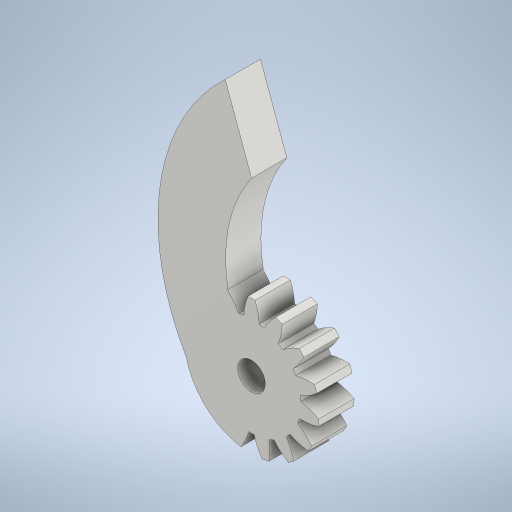
# Autodesk Inventor part: Spur Gear1
Saved by Autodesk Inventor 2024 (Build 280153000, 153)
## iProperties
CustomPartVersion: 1
Created: 2023-09-24
Part Number: Spur Gear1
Material: Steel
Document SubType Name: Modeling
Designer: jebes windows
Categories: <?xml version="1.0" encoding="UTF-16"?> <MemberInstance><Categories><FamilyTemplate><FamilyTemplateParameter ValueType="xs:double" Id="1" ObjectReferenceKey="da_z" ObjectType="kUserParameterObject"/><FamilyTemplateParameter ValueType="xs:double" Id="2" ObjectReferenceKey="da_b" ObjectType="kUserParameterObject"/><FamilyTemplateParameter ValueType="xs:double" Id="3" ObjectReferenceKey="da_beta" ObjectType="kUserParameterObject"/><FamilyTemplateParameter ValueType="xs:double" Id="4" ObjectReferenceKey="da_da" ObjectType="kUserParameterObject"/><FamilyTemplateParameter ValueType="xs:double" Id="5" ObjectReferenceKey="da_aw" ObjectType="kUserParameterObject"/><FamilyTemplateParameter ValueType="xs:string" Id="6" ObjectReferenceKey="EAIAABAAAACIAQAAAAAAAIAAAAAAAAAA" ObjectType="83910656" SubObjectId="SurfaceGeometry"/></FamilyTemplate><ParamToTemplateMap><ParamToTemplate CategoryParameter="//CategoryParameter[@InternalName='046C89C9-8512-4d59-83FE-43B91F4F132A']" TemplateParameter="1"/><ParamToTemplate CategoryParameter="//CategoryParameter[@InternalName='2552DF32-E462-4b46-AEBF-C6C7768E72AC']" TemplateParameter="2"/><ParamToTemplate CategoryParameter="//CategoryParameter[@InternalName='C9EE641D-15FC-4fae-A226-E94C4372FDD7']" TemplateParameter="3"/><ParamToTemplate><ParamToTemplate CategoryParameter="//CategoryParameter[@InternalName='00B6519A-459B-49c7-AD84-2E56D39A5744']" ConstantValue="0.000000"/></ParamToTemplate><ParamToTemplate><ParamToTemplate CategoryParameter="//CategoryParameter[@InternalName='04B31F0E-C7A6-4894-AA32-9629BEFACF47']" ConstantValue="1.000000"/></ParamToTemplate><ParamToTemplate><ParamToTemplate CategoryParameter="//CategoryParameter[@InternalName='43CBEC2E-7847-49e7-A936-2F7889FCB2D9']" ConstantValue="0.250000"/></ParamToTemplate><ParamToTemplate><ParamToTemplate CategoryParameter="//CategoryParameter[@InternalName='B1EFC894-105D-4ebd-86BF-FA20ED196853']" ConstantValue="0.302500"/></ParamToTemplate><ParamToTemplate><ParamToTemplate CategoryParameter="//CategoryParameter[@InternalName='51175063-3D10-4879-93E8-6246FE8B403D']" ConstantValue="2060000000.000000"/></ParamToTemplate><ParamToTemplate><ParamToTemplate CategoryParameter="//CategoryParameter[@InternalName='A3A52E27-4454-46a9-B0BD-C932399B70AF']" ConstantValue="0.300000"/></ParamToTemplate><ParamToTemplate><ParamToTemplate CategoryParameter="//CategoryParameter[@InternalName='91B76062-C214-41d9-B1B9-14D2AB99603D']" ConstantValue="0.150000"/></ParamToTemplate><ParamToTemplate><ParamToTemplate CategoryParameter="//CategoryParameter[@InternalName='374E806E-8B8A-4dda-A9AA-1039D6500AD2']" ConstantValue="6.666667"/></ParamToTemplate><ParamToTemplate><ParamToTemplate CategoryParameter="//CategoryParameter[@InternalName='2D373A89-B862-43d6-8D0B-0CBF12AB9F6C']" ConstantValue="0.349066"/></ParamToTemplate><ParamToTemplate CategoryParameter="//CategoryParameter[@InternalName='37777632-D6A2-4fac-9D53-DB8ACD95C989']" TemplateParameter="4"/><ParamToTemplate CategoryParameter="//CategoryParameter[@InternalName='FD1017F1-B727-4f7e-9707-0F86F1FF9423']" TemplateParameter="5"/><ParamToTemplate><ParamToTemplate CategoryParameter="//CategoryParameter[@InternalName='9E1B4470-B2D3-4ff1-B813-535BB4CDF51A']" ConstantValue="3520000.000000"/></ParamToTemplate><ParamToTemplate><ParamToTemplate CategoryParameter="//CategoryParameter[@InternalName='F8452263-BFF6-458c-9FB1-07C4B99E95CD']" ConstantValue="11400000.000000"/></ParamToTemplate><ParamToTemplate><ParamToTemplate CategoryParameter="//CategoryParameter[@InternalName='3E3BB259-FD49-497f-8171-6EBC954A3479']" ConstantValue="2.000000"/></ParamToTemplate><ParamToTemplate CategoryParameter="//CategoryParameter[@InternalName='27C3BAF2-7550-4e4b-AE2C-0DB134B7D9B7']" TemplateParameter="6"/></ParamToTemplateMap><Category DisplayName="Gear" InternalName="DC85795E-93AB-48d5-8EEE-5A27447B64BD" Mnemonic="Gear"><CategoryParameter DisplayName="z" InternalName="046C89C9-8512-4d59-83FE-43B91F4F132A" Mnemonic="z"/><CategoryParameter DisplayName="b" InternalName="2552DF32-E462-4b46-AEBF-C6C7768E72AC" Mnemonic="b"/><CategoryParameter DisplayName="||b|" InternalName="C9EE641D-15FC-4fae-A226-E94C4372FDD7" Mnemonic="beta"/><CategoryParameter DisplayName="x" InternalName="00B6519A-459B-49c7-AD84-2E56D39A5744" Mnemonic="x"/><CategoryParameter DisplayName="a*" InternalName="04B31F0E-C7A6-4894-AA32-9629BEFACF47" Mnemonic="a"/><CategoryParameter DisplayName="c*" InternalName="43CBEC2E-7847-49e7-A936-2F7889FCB2D9" Mnemonic="c"/><CategoryParameter DisplayName="r|.f|*" InternalName="B1EFC894-105D-4ebd-86BF-FA20ED196853" Mnemonic="rf"/><CategoryParameter DisplayName="E" InternalName="51175063-3D10-4879-93E8-6246FE8B403D" Mnemonic="E"/><CategoryParameter DisplayName="||m|" InternalName="A3A52E27-4454-46a9-B0BD-C932399B70AF" Mnemonic="mi"/><Category DisplayName="SpurGear" InternalName="26C5A22E-A91E-4dfd-A3B3-23CCAFAE1764" Mnemonic="SpurGear"><CategoryParameter DisplayName="m" InternalName="91B76062-C214-41d9-B1B9-14D2AB99603D" Mnemonic="m"/><CategoryParameter DisplayName="P" InternalName="374E806E-8B8A-4dda-A9AA-1039D6500AD2" Mnemonic="PP"/><CategoryParameter DisplayName="||a|" InternalName="2D373A89-B862-43d6-8D0B-0CBF12AB9F6C" Mnemonic="alpha"/><CategoryParameter DisplayName="d|.a|" InternalName="37777632-D6A2-4fac-9D53-DB8ACD95C989" Mnemonic="da"/><CategoryParameter DisplayName="a|.w|" InternalName="FD1017F1-B727-4f7e-9707-0F86F1FF9423" Mnemonic="aw"/><CategoryParameter DisplayName="||s||.Flim|" InternalName="9E1B4470-B2D3-4ff1-B813-535BB4CDF51A" Mnemonic="sFlim"/><CategoryParameter DisplayName="||s||.Hlim|" InternalName="F8452263-BFF6-458c-9FB1-07C4B99E95CD" Mnemonic="sHlim"/><CategoryParameter DisplayName="type" InternalName="3E3BB259-FD49-497f-8171-6EBC954A3479" Mnemonic="type"/><CategoryParameter DisplayName="PitchDiameter" InternalName="27C3BAF2-7550-4e4b-AE2C-0DB134B7D9B7" Mnemonic="IDS_PITCHDIAM"/></Category></Category></Categories></MemberInstance>
Density: 1 g/cm^3
Appearance: Steel
Author: jebes windows
## iProperties of the stored document Spur Gear11_3DPrint.ipt
Created: 2023-09-24
Part Number: Spur Gear11_3DPrint
Material: Generic
Document SubType Name: Modeling
Designer: jebes windows
Density: 1 g/cm^3
Appearance: Default
Author: jebes windows
Autodesk Inventor part; units mm, degrees
sketch "Sketch1" plane through (0, 0, 0) normal (0, 0, 1) x (1, 0, 0)
  circle A0 centre (0, 0) radius 12.7464
  dimension "d0" = 25.4929
  constraints: 1 centre point
  measures "d0" diameter of A0
extrude "Extrusion1" add sketch "Sketch1" along normal blind 6.6667
ref_plane "Work Plane2" through (0, 0, 3.3333) normal (0, 0, 1) x (1, 0, 0)
sketch "Sketch2" plane through (0, 0, 0) normal (0, 0, -1) x (-1, 0, 0)
  circle A0 centre (0, 0) radius 12.7464 projected
  circle A1 centre (0, 0) radius 11.25
  dimension "d3" = 22.5
  constraints: 1 centre point, 1 coincident
  measures "d3" diameter of A1
surface extrude "Pitch Diameter" sketch "Sketch2" against normal through all shown no curves A1
ref_plane "Work Plane8" through (0, 0, 0) normal (0.9781476, 0.2079117, 0) x (0, 0, 1)
ref_plane "Work Plane9" through (0, 0, 0) normal (1, 0, 0) x (0, 1, 0)
spur gear teeth "Spur Gear" teeth 15 pitch diameter 22.5 tip diameter 25.4929 root diameter 18.75 face width 10 start plane through (0, 0, 0) normal (0, 0, -1) x (-1, 0, 0)
sketch "Sketch3" plane through (0, 0, 0) normal (0, 0, -1) x (-1, 0, 0)
  circle A0 centre (0, 0) radius 2.6
  dimension "d49" = 5.2
  constraints: 1 centre point, 1 coincident
  measures "d49" diameter of A0
extrude "Extrusion2" cut sketch "Sketch3" against normal blind 10
sketch "Sketch7" plane through (0, 0, 6.6667) normal (0, 0, 1) x (1, 0, 0)
  circle A0 centre (0, 0) radius 2.6 projected
  line L0 (0, 0) -> (0, 50)
  arc A1 (0.6671, 12.729) -> (-0.6671, 12.729) centre (0, 0) ccw projected
  circle A2 centre (22.118, 16.88) radius 27.0188
  circle A3 centre (22.118, 16.88) radius 39.8269
  line L1 (0, 32.3981) -> (-4.9763, 46.0704)
  circle A4 centre (0, 0) radius 12.7464
  circle A5 centre (0, 0) radius 2.6 projected
  arc A6 (-5.7868, 11.3571) -> (-5.106, 7.8625) centre (4.8126, 11.6083) ccw projected
  arc A7 (-5.106, 7.8625) -> (-5.8999, 7.2857) centre (0, 0) ccw projected
  arc A8 (-5.8999, 7.2857) -> (-9.0131, 9.0131) centre (-12.5273, -0.9898) ccw projected
  arc A9 (-9.0131, 9.0131) -> (-9.9058, 8.0216) centre (0, 0) ccw projected
  arc A10 (-9.9058, 8.0216) -> (-7.8625, 5.106) centre (-0.325, 12.5622) ccw projected
  arc A11 (-7.8625, 5.106) -> (-8.3532, 4.2562) centre (0, 0) ccw projected
  arc A12 (-8.3532, 4.2562) -> (-11.8998, 4.5679) centre (-11.0417, -5.9996) ccw projected
  arc A13 (-11.8998, 4.5679) -> (-12.3121, 3.299) centre (0, 0) ccw projected
  arc A14 (-12.3121, 3.299) -> (-9.2596, 1.4666) centre (-5.4064, 11.3439) ccw projected
  arc A15 (-9.2596, 1.4666) -> (-9.3622, 0.4906) centre (0, 0) ccw projected
  arc A16 (-9.3622, 0.4906) -> (-12.729, -0.6671) centre (-7.6468, -9.972) ccw projected
  arc A17 (-12.729, -0.6671) -> (-12.5895, -1.994) centre (0, 0) ccw projected
  arc A18 (-12.5895, -1.994) -> (-9.0556, -2.4264) centre (-9.553, 8.1642) ccw projected
  arc A19 (-9.0556, -2.4264) -> (-8.7523, -3.3597) centre (0, 0) ccw projected
  arc A20 (-8.7523, -3.3597) -> (-11.3571, -5.7868) centre (-2.9298, -12.2201) ccw projected
  arc A21 (-11.3571, -5.7868) -> (-10.6901, -6.9422) centre (0, 0) ccw projected
  arc A22 (-10.6901, -6.9422) -> (-7.2857, -5.8999) centre (-12.0478, 3.5728) ccw projected
  arc A23 (-7.2857, -5.8999) -> (-6.6291, -6.6291) centre (0, 0) ccw projected
  arc A24 (-6.6291, -6.6291) -> (-8.0216, -9.9058) centre (2.2939, -12.3552) ccw projected
  arc A25 (-8.0216, -9.9058) -> (-6.9422, -10.6901) centre (0, 0) ccw projected
  arc A26 (-6.9422, -10.6901) -> (-4.2562, -8.3532) centre (-12.4594, -1.6364) ccw projected
  arc A27 (-4.2562, -8.3532) -> (-3.3597, -8.7523) centre (0, 0) ccw projected
  arc A28 (-3.3597, -8.7523) -> (-3.299, -12.3121) centre (7.1209, -10.3541) ccw projected
  arc A29 (-3.299, -12.3121) -> (-1.994, -12.5895) centre (0, 0) ccw projected
  arc A30 (-1.994, -12.5895) -> (-0.4906, -9.3622) centre (-10.7166, -6.5626) ccw projected
  arc A31 (-0.4906, -9.3622) -> (0.4906, -9.3622) centre (0, 0) ccw projected
  arc A32 (0.4906, -9.3622) -> (1.994, -12.5895) centre (10.7166, -6.5626) ccw projected
  arc A33 (1.994, -12.5895) -> (3.299, -12.3121) centre (0, 0) ccw projected
  arc A34 (3.299, -12.3121) -> (3.3597, -8.7523) centre (-7.1209, -10.3541) ccw projected
  arc A35 (3.3597, -8.7523) -> (4.2562, -8.3532) centre (0, 0) ccw projected
  arc A36 (4.2562, -8.3532) -> (6.9422, -10.6901) centre (12.4594, -1.6364) ccw projected
  arc A37 (6.9422, -10.6901) -> (8.0216, -9.9058) centre (0, 0) ccw projected
  arc A38 (8.0216, -9.9058) -> (6.6291, -6.6291) centre (-2.2939, -12.3552) ccw projected
  arc A39 (6.6291, -6.6291) -> (7.2857, -5.8999) centre (0, 0) ccw projected
  arc A40 (7.2857, -5.8999) -> (10.6901, -6.9422) centre (12.0478, 3.5728) ccw projected
  arc A41 (10.6901, -6.9422) -> (11.3571, -5.7868) centre (0, 0) ccw projected
  arc A42 (11.3571, -5.7868) -> (8.7523, -3.3597) centre (2.9298, -12.2201) ccw projected
  arc A43 (8.7523, -3.3597) -> (9.0556, -2.4264) centre (0, 0) ccw projected
  arc A44 (9.0556, -2.4264) -> (12.5895, -1.994) centre (9.553, 8.1642) ccw projected
  arc A45 (12.5895, -1.994) -> (12.729, -0.6671) centre (0, 0) ccw projected
  arc A46 (12.729, -0.6671) -> (9.3622, 0.4906) centre (7.6468, -9.972) ccw projected
  arc A47 (9.3622, 0.4906) -> (9.2596, 1.4666) centre (0, 0) ccw projected
  arc A48 (9.2596, 1.4666) -> (12.3121, 3.299) centre (5.4064, 11.3439) ccw projected
  arc A49 (12.3121, 3.299) -> (11.8998, 4.5679) centre (0, 0) ccw projected
  arc A50 (11.8998, 4.5679) -> (8.3532, 4.2562) centre (11.0417, -5.9996) ccw projected
  arc A51 (8.3532, 4.2562) -> (7.8625, 5.106) centre (0, 0) ccw projected
  arc A52 (7.8625, 5.106) -> (9.9058, 8.0216) centre (0.325, 12.5622) ccw projected
  arc A53 (9.9058, 8.0216) -> (9.0131, 9.0131) centre (0, 0) ccw projected
  arc A54 (9.0131, 9.0131) -> (5.8999, 7.2857) centre (12.5273, -0.9898) ccw projected
  arc A55 (5.8999, 7.2857) -> (5.106, 7.8625) centre (0, 0) ccw projected
  arc A56 (5.106, 7.8625) -> (5.7868, 11.3571) centre (-4.8126, 11.6083) ccw projected
  arc A57 (5.7868, 11.3571) -> (4.5679, 11.8998) centre (0, 0) ccw projected
  arc A58 (4.5679, 11.8998) -> (2.4264, 9.0556) centre (11.8469, 4.1911) ccw projected
  arc A59 (2.4264, 9.0556) -> (1.4666, 9.2596) centre (0, 0) ccw projected
  arc A60 (1.4666, 9.2596) -> (0.6671, 12.729) centre (-9.118, 8.6473) ccw projected
  arc A61 (0.6671, 12.729) -> (-0.6671, 12.729) centre (0, 0) ccw projected
  arc A62 (-0.6671, 12.729) -> (-1.4666, 9.2596) centre (9.118, 8.6473) ccw projected
  arc A63 (-1.4666, 9.2596) -> (-2.4264, 9.0556) centre (0, 0) ccw projected
  arc A64 (-2.4264, 9.0556) -> (-4.5679, 11.8998) centre (-11.8469, 4.1911) ccw projected
  arc A65 (-4.5679, 11.8998) -> (-5.7868, 11.3571) centre (0, 0) ccw projected
  point P0 (0, 12.7464)
  point P1 (-4.4465, 11.9457)
  point P2 (-12.3854, -3.0122)
  point P3 (-8.0216, -9.9058)
  point P4 (-10.6901, -6.9422)
  point P5 (-12.5895, -1.994)
  point P6 (-11.3571, -5.7868)
  point P7 (-12.3121, 3.299)
  point P8 (-12.729, -0.6671)
  point P9 (-9.9058, 8.0216)
  point P10 (-11.8998, 4.5679)
  point P11 (-5.7868, 11.3571)
  point P12 (-9.0131, 9.0131)
  point P13 (-6.7426, -10.5654)
  point P14 (-6.1736, -11.1516)
  point P15 (-3.299, -12.3121)
  point P16 (-6.9422, -10.6901)
  dimension "d68" = 54.0377
  dimension "d71" = 79.6539
  dimension "d64" = 50
  dimension "d69" = 22.118
  dimension "d70" = 16.88
  dimension "d72" = 20
  constraints: 4 end point, 2 coincident, 1 point on circle, 1 point on line, 1 vertical, 9 other
  measures "d64" distance of L0.start L0.end
  measures "d69" horizontal distance of point (0, 0) point (22.118, 16.88)
  measures "d70" vertical distance of point (0, 0) point (22.118, 16.88)
  measures "d72" angle of L0 L1
extrude "Extrusion4" add sketch "Sketch7" against normal up to surface (6.6667 mm away) contours A2 A4 A3 L1 | A6 A7 A8 A4 | A4 A18 A19 A20 A3 | A3 A20 A4 | A4 A26 A3 | A3 A26 A27 A28 A4 | A10 A11 A12 A4 | A22 A23 A24 A3 | A3 A24 A4 A22 | A4 A14 A15 A16
equation "\"d0\" = da_da"
equation "\"d1\" = 0.666667 * da_b"
equation "\"d3\" = da_d"
equation "\"d16\" = da_aw"
equation "\"d43\" = da_aw"
equation "\"d46\" = da_aw"
equation "\"da_da\" = 25.492855"
equation "\"da_b\" = 10"
equation "\"da_d\" = 22.5"
equation "\"da_aw\" = 23.4"
body "Solid1"
body "Srf1"
